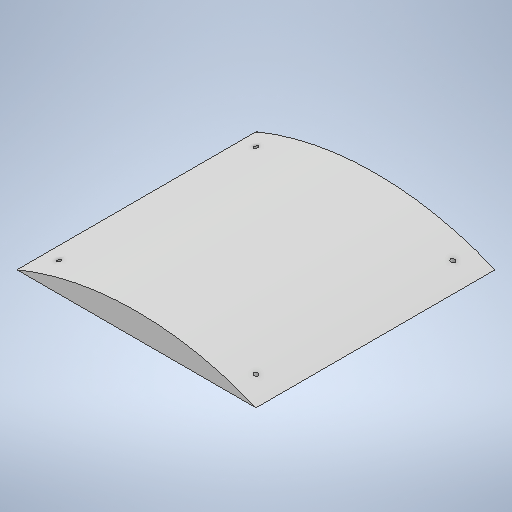
# Autodesk Inventor part: TopHead
Saved by Autodesk Inventor 2025 (Build 290162000, 162)
## iProperties
Created: 2025-09-02
Part Number: TopHead
Material: Generic
Document SubType Name: Modeling
Designer: wangb
Density: 1 g/cm^3
Appearance: Default
Author: wangb
Autodesk Inventor part; units mm, degrees
ref_plane "YZ Plane" through (0, 0, 0) normal (1, 0, 0) x (0, 1, 0)
ref_plane "XZ Plane" through (0, 0, 0) normal (0, 1, 0) x (-1, 0, 0)
ref_plane "XY Plane" through (0, 0, 0) normal (0, 0, 1) x (1, 0, 0)
sketch "Sketch1" plane through (0, 0, 0) normal (0, 0, 1) x (1, 0, 0)
  arc A0 (76.5789, 0) -> (-8.4211, 0) centre (34.0789, -102.0754) ccw
  line L0 (-8.4211, 0) -> (76.5789, 0)
  point P0 (0, 0)
  dimension "d0" = 85
  constraints: 2 end point, 2 point on circle, 1 centre point, 1 horizontal
  measures "d0" distance of L0.start L0.end
extrude "Extrusion1" add sketch "Sketch1" along normal blind 85
sketch "Sketch2" plane through (-8.4211, 0, 0) normal (0, -1, 0) x (1, 0, 0)
  circle A0 centre (7.5, 77.5) radius 0.75
  circle A1 centre (7.5, 7.5) radius 0.75
  circle A2 centre (77.5, 77.5) radius 0.75
  circle A3 centre (77.5, 7.5) radius 0.75
  line L0 (0, 85) -> (85, 85) projected
  line L1 (0, 0) -> (85, 0) projected
  line L2 (85, 0) -> (85, 85) projected
  point P0 (8.4211, 0)
  point P1 (36.7967, 13.095)
  dimension "d3" = 1.5
  dimension "d4" = 1.5
  dimension "d5" = 1.5
  dimension "d6" = 1.5
  dimension "d7" = 70
  dimension "d8" = 7.5
  dimension "d9" = 7.5
  dimension "d10" = 70
  dimension "d11" = 70
  dimension "d12" = 70
  dimension "d13" = 7.5
  dimension "d14" = 7.5
  constraints: 4 centre point
  measures "d3" diameter of A0
  measures "d4" diameter of A1
  measures "d5" diameter of A2
  measures "d6" diameter of A3
  measures "d7" distance of A1.centre A0.centre
  measures "d8" distance from line of L0 A0.centre
  measures "d9" distance from line of L1 A1.centre
  measures "d10" distance of A0.centre A2.centre
  measures "d11" distance of A1.centre A3.centre
  measures "d12" distance of A3.centre A2.centre
  measures "d13" distance from line of L1 A3.centre
  measures "d14" distance from line of L2 A2.centre
extrude "Extrusion2" cut sketch "Sketch2" against normal blind 85
body "Solid1"
